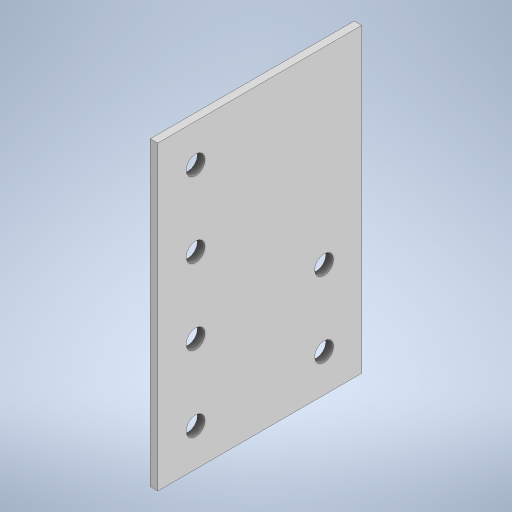
# Autodesk Inventor part: H-Connector_2020
Saved by Autodesk Inventor 2024 (Build 280153000, 153)
## iProperties
Created: 2025-12-25
Part Number: H-Connector_2020
Material: Generic
Document SubType Name: Modeling
Designer: schar
Density: 1 g/cm^3
Appearance: Default
Author: schar
Autodesk Inventor part; units mm, degrees
ref_plane "YZ Plane" through (0, 0, 0) normal (1, 0, 0) x (0, 1, 0)
ref_plane "XZ Plane" through (0, 0, 0) normal (0, 1, 0) x (-1, 0, 0)
ref_plane "XY Plane" through (0, 0, 0) normal (0, 0, 1) x (1, 0, 0)
sketch "Sketch1" plane through (0, 0, 0) normal (1, 0, 0) x (0, 1, 0)
  line L0 (0, 0) -> (-40, 0)
  line L1 (-40, 0) -> (-40, -54.112)
  line L2 (-40, -54.112) -> (0, -54.112)
  line L3 (0, -54.112) -> (0, 0)
  line L4 (-40, -54.112) -> (-40, -44.112)
  line L5 (-40, -44.112) -> (-30, -44.112)
  line L6 (-40, 0) -> (-40, -10)
  line L7 (-40, -10) -> (-30, -10)
  line L8 (0, -10) -> (-10, -10)
  circle A0 centre (-10, -10) radius 2.5
  circle A1 centre (-30, -44.112) radius 2.5
  circle A2 centre (-30, -10) radius 2.5
  line L9 (-40, 0) -> (-60, 0)
  line L10 (-60, 0) -> (-60, -54.112)
  line L11 (-60, -54.112) -> (-40, -54.112)
  line L12 (-40, -54.112) -> (-40, 0)
  line L13 (0, 0) -> (20, 0)
  line L14 (20, 0) -> (20, -54.112)
  line L15 (20, -54.112) -> (0, -54.112)
  line L16 (0, -54.112) -> (0, 0)
  circle A3 centre (10, -10) radius 2.5
  circle A4 centre (-50, -44.112) radius 2.5
  circle A5 centre (-50, -10) radius 2.5
  line L17 (0, -54.112) -> (0, -44.112)
  line L18 (0, -44.112) -> (-10, -44.112)
  circle A6 centre (-10, -44.112) radius 2.5
  circle A7 centre (10, -44.112) radius 2.5
  dimension "d0" = 40
  dimension "d1" = 54.112
  dimension "d2" = 10
  dimension "d3" = 10
  dimension "d4" = 10
  dimension "d5" = 10
  dimension "d6" = 5
  dimension "d8" = 5
  dimension "d9" = 5
  dimension "d10" = 20
  dimension "d11" = 20
  dimension "d14" = 10
  dimension "d15" = 10
  dimension "d16" = 5
  constraints: 38 end point, 8 centre point, 6 parallel, 6 perpendicular, 5 point on line, 4 coincident, 4 horizontal, 4 symmetric about line, 4 other
  measures "d0" distance of L2.end L1.end
  measures "d1" distance of L1.end L0.end
  measures "d2" distance of L1.end L4.end
  measures "d3" distance of L4.end L5.end
  measures "d4" distance of L0.end L6.end
  measures "d5" distance of L8.start L8.end
  measures "d6" diameter of A0
  measures "d8" diameter of A1
  measures "d9" diameter of A2
  measures "d10" distance of L11.end L10.end
  measures "d11" distance of L14.end L15.end
  measures "d14" distance of L15.end L17.end
  measures "d15" distance of L17.end L18.end
  measures "d16" diameter of A6
extrude "Extrusion1" add sketch "Sketch1" along normal blind 2 contours L3 L2 L1 L0 | L13 L14 L15 L3 | L1 L11 L10 L9 | A6 | A7
body "Solid1"
